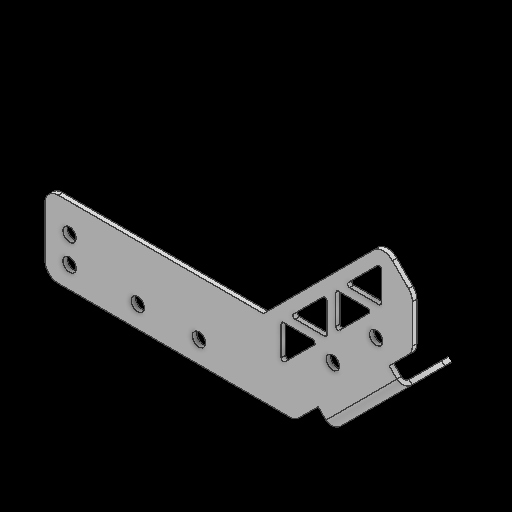
# Autodesk Inventor part: Part1
Saved by Autodesk Inventor 2025.2 (Build 292293000, 293)
## iProperties
Created: 2026-06-08
Part Number: Part1
Material: Generic
Document SubType Name: Sheet Metal
Designer: valer
Density: 1 g/cm^3
Sheet Metal Rule: Default
Appearance: Default
Author: valer
Autodesk Inventor part; units mm, degrees
ref_plane "YZ Plane" through (0, 0, 0) normal (1, 0, 0) x (0, 1, 0)
ref_plane "XZ Plane" through (0, 0, 0) normal (0, 1, 0) x (-1, 0, 0)
ref_plane "XY Plane" through (0, 0, 0) normal (0, 0, 1) x (1, 0, 0)
sketch "Sketch1" plane through (0, 0, 0) normal (0, 0, 1) x (1, 0, 0)
  line L0 (-38.75, 11.0048) -> (-38.75, 0.5861)
  line L1 (38.75, 17.1008) -> (-38.75, 17.1008)
  arc A0 (-38.75, 0.5861) -> (-36.9926, -3.6566) centre (-32.75, 0.5861) ccw
  line L2 (-24.5074, -16.1418) -> (-36.9926, -3.6566)
  arc A1 (-24.5074, -16.1418) -> (-20.2647, -17.8992) centre (-20.2647, -11.8992) ccw
  line L3 (20.2647, -17.8992) -> (-20.2647, -17.8992)
  arc A2 (20.2647, -17.8992) -> (24.5074, -16.1418) centre (20.2647, -11.8992) ccw
  line L4 (36.9926, -3.6566) -> (24.5074, -16.1418)
  arc A3 (36.9926, -3.6566) -> (38.75, 0.5861) centre (32.75, 0.5861) ccw
  line L5 (38.75, 11.0048) -> (38.75, 0.5861)
  line L6 (38.75, 11.0048) -> (-38.75, 11.0048)
  line L7 (-38.75, 0.5861) -> (-38.75, 11.0048)
  line L8 (93.5508, 71.9016) -> (38.75, 17.1008)
  arc A4 (50.4277, 5.4231) -> (54.6703, 3.6658) centre (54.6703, 9.6658) ccw
  line L9 (72.3272, 3.6658) -> (54.6703, 3.6658)
  arc A5 (72.3272, 3.6658) -> (76.5698, 5.4231) centre (72.3272, 9.6658) ccw
  line L10 (105.2284, 34.0818) -> (76.5698, 5.4231)
  arc A6 (105.2284, 34.0818) -> (106.9858, 38.3244) centre (100.9858, 38.3244) ccw construction
  line L11 (106.9858, 55.9813) -> (106.9858, 38.3244)
  arc A7 (106.9858, 55.9813) -> (105.2284, 60.2239) centre (100.9858, 55.9813) ccw
  line L12 (97.8613, 67.591) -> (105.2284, 60.2239)
  line L13 (97.8613, 67.591) -> (43.0605, 12.7903)
  line L14 (50.4277, 5.4231) -> (43.0605, 12.7903)
  line L15 (93.5508, 71.9016) -> (97.8613, 67.591)
  line L16 (20.2647, -17.8992) -> (53.2475, -17.8992)
  line L17 (53.2475, -17.8992) -> (76.5698, 5.4231)
  line L18 (105.2284, 34.0818) -> (106.9858, 35.8391)
  line L19 (106.9858, 35.8391) -> (106.9858, 38.3244)
  line L20 (72.3272, 3.6658) -> (74.8124, 3.6658)
  line L21 (74.8124, 3.6658) -> (76.5698, 5.4231)
  line L22 (-61.25, -11.8992) -> (-61.25, 13.1008)
  arc A8 (-61.25, -11.8992) -> (-55.25, -17.8992) centre (-55.25, -11.8992) ccw
  line L23 (-38.75, 17.1008) -> (-61.25, 17.1008)
  line L24 (-55.25, -17.8992) -> (-20.2647, -17.8992)
  line L25 (-61.25, 17.1008) -> (-61.25, 13.1008)
  point P0 (0, 0)
extrude "Plate1" add sketch "Sketch1" along normal blind 2.032
fillet "Fillet3" radius 6 4 edges at (106.9858, 35.8391, 1.016) (53.2475, -17.8992, 1.016) (93.5508, 71.9016, 1.016) (-61.25, 17.1008, 1.016)
sketch "Sketch3" plane through (0, 0, 2.032) normal (0, 0, 1) x (1, 0, 0)
  line L0 (106.9858, 35.8391) -> (53.2475, -17.8992)
  line L1 (96.3792, 25.2325) -> (99.9147, 21.697)
  line L2 (99.9147, 21.697) -> (67.3896, -10.8281)
  line L3 (67.3896, -10.8281) -> (63.8541, -7.2926)
  point P0 (0, 0)
  dimension "d6" = 15
  dimension "d7" = 15
  dimension "d8" = 5
  measures "d6" distance from line of L0.start L1
  measures "d7" distance from line of L0.end L3
  measures "d8" distance between parallel lines of L0 L2
sheet face with bend "Face2" sketch "Sketch3" thickness 2.032 toward (0, 0, -1) bend radius 2.032
bend "Bend1"
sketch "Sketch4" plane through (101.3516, 20.2601, -2.032) normal (0.7071068, -0.7071068, 0) x (0.7071068, 0.7071068, 0)
  line L0 (-45.9975, 0) -> (0, 0)
  line L1 (0, 0) -> (0, 20.936)
  line L2 (0, 20.936) -> (-45.9975, 20.936)
  line L3 (-45.9975, 20.936) -> (-45.9975, 0)
  constraints: 6 end point, 1 horizontal, 1 perpendicular, 1 vertical
edge flange "Flange1" height 25 angle 90 thickness 2.032 bend radius 2.032 thickness toward (0.7071068, -0.7071068, 0) relief tear relief width 2.032 relief depth 1.016 edges at (83.6522, 5.4344, 2.032) wall of the first edge with corners at (68.8265, -12.265, -2.032) (101.3516, 20.2601, -2.032) (101.3516, 20.2601, -22.968) (68.8265, -12.265, -22.968)
bend "Bend2"
corner "Corner1"
fillet "Fillet4" radius 6 2 edges at (102.07, 19.5417, -22.968) (69.5449, -12.9834, -22.968)
sketch "Sketch7" plane through (0, 0, 2.032) normal (0, 0, 1) x (1, 0, 0)
  circle A0 centre (9.2378, -7.8992) radius 3
  circle A1 centre (-18.7622, -7.8992) radius 3
  point P0 (0, 0)
  constraints: 2 centre point, 4 other
extrude "Cut4" cut sketch "Sketch7" against normal through all
sketch "Sketch8" plane through (0, 0, 2.032) normal (0, 0, 1) x (1, 0, 0)
  circle A0 centre (90.3602, 33.3556) radius 3
  circle A1 centre (70.5612, 13.5566) radius 3
  point P0 (0, 0)
  constraints: 2 centre point, 4 other
extrude "Cut5" cut sketch "Sketch8" against normal through all
sketch "Sketch10" plane through (102.7884, 18.8233, -2.032) normal (0.7071068, -0.7071068, 0) x (-0.7071068, -0.7071068, 0)
  arc A0 (45.9975, 14.936) -> (39.9975, 20.936) centre (39.9975, 14.936) ccw construction
  arc A1 (45.9975, 14.936) -> (39.9975, 20.936) centre (39.9975, 14.936) ccw construction
  line L0 (39.9975, 20.936) -> (6, 20.936) construction
  arc A2 (6, 20.936) -> (0, 14.936) centre (6, 14.936) ccw construction
  line L1 (0, 0) -> (0, 14.936) construction
  line L2 (0, 0) -> (45.9975, 0) construction
  line L3 (45.9975, 0) -> (45.9975, 14.936) construction
  line L4 (0, 0) -> (0, 14.936) construction
  line L5 (0, 12.936) -> (45.9975, 12.936) construction
  line L6 (45.9975, 0) -> (45.9975, 14.936) construction
  circle A3 centre (37.9975, 12.936) radius 3
  line L7 (0, 0) -> (45.9975, 0) projected
  line L8 (22.9987, 0) -> (22.9987, 20.936) construction
  circle A4 centre (8, 12.936) radius 3
  point P0 (85.9925, -2.032)
  dimension "d54" = 8
  dimension "d55" = 6
  dimension "d56" = 8
  constraints: 4 end point, 3 point on line, 2 centre point, 2 midpoint, 1 parallel, 1 symmetric about line, 1 other
  measures "d54" distance between parallel lines of L5 L0
  measures "d55" diameter of A3
  measures "d56" distance from line of L6 A3.centre
extrude "Cut7" cut sketch "Sketch10" against normal through all
sketch "Sketch12" plane through (0, 0, 2.032) normal (0, 0, 1) x (1, 0, 0)
  circle A0 centre (70.5612, 13.5566) radius 3 projected
  circle A1 centre (90.3602, 33.3556) radius 3 projected
  circle A2 centre (9.2378, -7.8992) radius 3 projected
  circle A3 centre (-18.7622, -7.8992) radius 3 projected
  arc A4 (97.7934, 67.6589) -> (89.3081, 67.6589) centre (93.5508, 63.4163) ccw projected
  line L0 (38.75, 17.1008) -> (89.3081, 67.6589) projected
  line L1 (-55.25, 17.1008) -> (38.75, 17.1008) projected
  line L2 (50.7622, -17.8992) -> (-55.25, -17.8992) projected
  arc A5 (50.7622, -17.8992) -> (55.0048, -16.1418) centre (50.7622, -11.8992) ccw projected
  line L3 (63.8541, -7.2926) -> (55.0048, -16.1418) projected
  line L4 (63.8541, -7.2926) -> (67.3896, -10.8281) projected
  line L5 (67.3896, -10.8281) -> (99.9147, 21.697) projected
  line L6 (99.9147, 21.697) -> (96.3792, 25.2325) projected
  arc A6 (105.2284, 34.0818) -> (106.9858, 38.3244) centre (100.9858, 38.3244) ccw projected
  line L7 (106.9858, 55.9813) -> (106.9858, 38.3244) projected
  arc A7 (106.9858, 55.9813) -> (105.2284, 60.2239) centre (100.9858, 55.9813) ccw projected
  line L8 (97.7934, 67.6589) -> (105.2284, 60.2239) projected
  line L9 (92.8437, 64.1234) -> (92.8437, 47.1528)
  line L10 (92.8437, 47.1528) -> (75.8731, 47.1528)
  line L11 (75.8731, 47.1528) -> (92.8437, 64.1234)
  line L12 (38.75, 17.1008) -> (89.3081, 67.6589) projected
  line L13 (92.8437, 47.1528) -> (84.3584, 55.6381) construction
  line L14 (75.8731, 47.1528) -> (71.8731, 43.1528) construction
  line L15 (71.8731, 43.1528) -> (88.8437, 43.1528)
  line L16 (88.8437, 43.1528) -> (92.8437, 47.1528) construction
  line L17 (71.8731, 43.1528) -> (71.8731, 26.1823)
  line L18 (71.8731, 26.1823) -> (88.8437, 43.1528)
  line L19 (71.8731, 43.1528) -> (80.3584, 34.6676) construction
  line L20 (50.9025, 22.1823) -> (67.8731, 22.1823)
  line L21 (67.8731, 22.1823) -> (67.8731, 39.1528)
  line L22 (67.8731, 39.1528) -> (50.9025, 22.1823)
  line L23 (67.8731, 22.1823) -> (59.3878, 30.6676) construction
  line L24 (46.9025, 18.1823) -> (46.9025, 1.2117)
  line L25 (46.9025, 18.1823) -> (63.8731, 18.1823)
  line L26 (63.8731, 18.1823) -> (46.9025, 1.2117)
  line L27 (46.9025, 18.1823) -> (55.3878, 9.697) construction
  line L28 (-61.25, -11.8992) -> (-61.25, 11.1008) projected
  arc A8 (-61.25, -11.8992) -> (-55.25, -17.8992) centre (-55.25, -11.8992) ccw projected
  line L29 (105.2284, 34.0818) -> (96.3792, 25.2325) projected
  arc A9 (-55.25, 17.1008) -> (-61.25, 11.1008) centre (-55.25, 11.1008) ccw projected
  point P0 (0, 0)
  dimension "d62" = 5
  dimension "d64" = 6
  dimension "d65" = 4
  constraints: 36 end point, 6 symmetric about line, 4 midpoint, 4 parallel, 2 perpendicular, 1 collinear, 1 horizontal, 1 point on line
  measures "d62" distance between parallel lines of L0 L11
  measures "d64" distance from line of L8 L9.start
  measures "d65" distance between parallel lines of L10 L15
extrude "Cut9" cut sketch "Sketch12" against normal through all contours L9 L10 L11 | L15 L18 L17 | L22 L21 L20 | L25 L26 L24
fillet "Fillet5" radius 1 12 edges at (92.8437, 64.1234, 1.016) (75.8731, 47.1528, 1.016) (92.8437, 47.1528, 1.016) (71.8731, 43.1528, 1.016) (71.8731, 26.1823, 1.016) (88.8437, 43.1528, 1.016) (67.8731, 39.1528, 1.016) (50.9025, 22.1823, 1.016) (67.8731, 22.1823, 1.016) (46.9025, 18.1823, 1.016) (63.8731, 18.1823, 1.016) (46.9025, 1.2117, 1.016)
sketch "Sketch13" plane through (0, 0, 2.032) normal (0, 0, 1) x (1, 0, 0)
  circle A0 centre (-50, 4.1008) radius 3
  circle A1 centre (-50, -7.8992) radius 3
  point P0 (0, 0)
  constraints: 2 centre point, 4 other
extrude "Cut10" cut sketch "Sketch13" against normal through all
equation "\"d48\" = Thickness"
equation "\"d50\" = Thickness"
equation "\"d57\" = Thickness"
equation "\"d66\" = Thickness"
equation "\"d69\" = Thickness"
equation "\"d0\" = Thickness"
equation "\"d9\" = BendRadius"
equation "\"d10\" = BendReliefWidth"
equation "\"d12\" = MinimumRemnant"
equation "\"d11\" = BendReliefDepth"
equation "\"d13\" = TransitionRadius"
equation "\"d14\" = BendReliefWidth"
equation "\"d15\" = BendReliefDepth"
equation "\"d16\" = MinimumRemnant"
equation "\"d17\" = TransitionRadius"
equation "\"d20\" = BendRadius"
equation "\"d21\" = CornerReliefSize"
equation "\"d22\" = GapSize"
equation "\"d23\" = JacobiRadiusSize"
equation "\"Thickness\" = 2.032"
equation "\"BendRadius\" = 2.032"
equation "\"BendReliefWidth\" = 2.032"
equation "\"MinimumRemnant\" = 4.064"
equation "\"BendReliefDepth\" = 1.016"
equation "\"TransitionRadius\" = 2.032"
equation "\"CornerReliefSize\" = 8.128"
equation "\"GapSize\" = 2.032"
equation "\"JacobiRadiusSize\" = 2.032"
body "Solid1"
